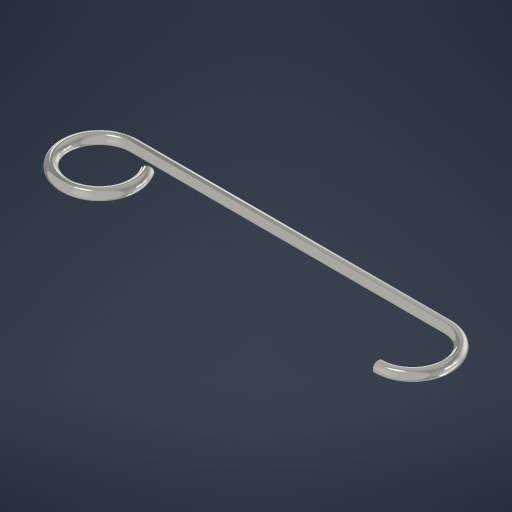
# Autodesk Inventor part: Gancho
Saved by Autodesk Inventor 2024 (Build 280153000, 153)
## iProperties
Created: 2015-11-26
Part Number: Gancho
Material: Acero
Document SubType Name: Modeling
Designer: H. Valenzuela B.
Density: 7.85 g/cm^3
Appearance: Plata
Author: H. Valenzuela B.
Autodesk Inventor part; units mm, degrees
ref_plane "YZ Plane" through (0, 0, 0) normal (1, 0, 0) x (0, 1, 0)
ref_plane "XZ Plane" through (0, 0, 0) normal (0, 1, 0) x (-1, 0, 0)
sketch "Boceto2" plane through (0, 0, 0) normal (1, 0, 0) x (0, 1, 0)
  circle A0 centre (13, 0) radius 2
  point P0 (0, 0)
  point P1 (13, 0)
  dimension "d4" = 4
  constraints: 1 centre point, 1 coincident
  measures "d4" diameter of A0
sketch "Boceto1" plane through (0, 0, 0) normal (0, 0, 1) x (1, 0, 0)
  line L0 (-68.813, 0) -> (68.813, 0) construction
  line L1 (49.5, 15) -> (-68.813, 15)
  arc A0 (49.5, -15) -> (49.5, 15) centre (49.5, 0) ccw
  line L2 (-68.813, 0) -> (68.813, 0) construction
  line L3 (49.5, 11) -> (-68.813, 11)
  arc A1 (49.5, -11) -> (49.5, 11) centre (49.5, 0) ccw
  line L4 (-68.813, 13) -> (49.5, 13)
  arc A2 (49.5, -13) -> (49.5, 13) centre (49.5, 0) ccw
  line L5 (49.5, -11) -> (49.5, -15)
  line L6 (-59.539, 5.9156) -> (-56.1667, 8.0667)
  arc A3 (-68.813, -11) -> (-59.539, 5.9156) centre (-68.813, 0) ccw
  arc A4 (-68.813, -13) -> (-57.8529, 6.9911) centre (-68.813, 0) ccw
  arc A5 (-68.813, 11) -> (-68.813, -11) centre (-68.813, 0) ccw
  arc A6 (-68.813, 13) -> (-68.813, -13) centre (-68.813, 0) ccw
  arc A7 (-68.813, 15) -> (-68.813, -15) centre (-68.813, 0) ccw
  arc A8 (-68.813, -15) -> (-56.1667, 8.0667) centre (-68.813, 0) ccw
  point P0 (0, 0)
  point P1 (64.5, 0)
  point P2 (-83.813, 0)
  dimension "d3" = 2
  dimension "d7" = 118.313
  dimension "d8" = 148.313
  dimension "d9" = 118.313
  dimension "d10" = 118.313
  constraints: 20 point on circle, 18 end point, 9 centre point, 3 midpoint, 2 tangent, 1 horizontal, 1 point on line, 1 other
  measures "d3" distance between parallel lines of L1 L4
  measures "d7" distance of L1.start L1.end
  measures "d8" distance of point (64.5, 0) point (-83.813, 0)
  measures "d9" distance of L4.start L4.end
  measures "d10" distance of L3.start L3.end
sweep "Barrido1" add profiles "Boceto2" path "Boceto1" path curves A4 A6 L4 A2
ref_plane "Plano de trabajo3" through (-68.813, 0, 0) normal (0, 0, -1) x (-1, 0, 0)
sketch "Boceto5" plane through (-68.813, 0, 0) normal (0, 0, -1) x (-1, 0, 0)
  arc A0 (-12.6463, 8.0667) -> (0, 15) centre (0, 0) ccw projected
  arc A1 (-118.313, 11) -> (-118.313, -11) centre (-118.313, 0) ccw projected
  arc A2 (-118.313, 15) -> (-118.313, -15) centre (-118.313, 0) ccw projected
  point P0 (-68.813, 0)
  point P1 (-110, 0)
  point P2 (-114, 0)
  point P3 (11, 0)
  point P4 (15, 0)
  point P5 (-129.313, 0)
  point P6 (-133.313, 0)
  constraints: 3 point on circle
